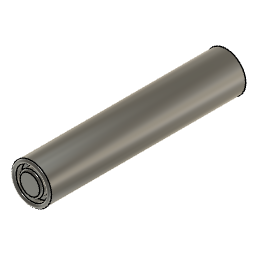
Shaker v1 (Autodesk Fusion 360 archive; units mm, degrees)
design "Shacker Pin Small"
Autodesk Fusion 360 part; units mm, degrees
sketch "Sketch1" plane through (0, 0, 0) normal (0, 1, 0) x (1, 0, 0)
  circle A0 centre (0, 0) radius 5
  dimension "d1" = 10
  constraint coincident A0.centre origin
  measures "d1" diameter of A0
extrude "Extrude1" add sketch "Sketch1" along normal blind 50
sketch "Sketch2" plane through (0, 0, 0) normal (0, -1, 0) x (1, 0, 0)
  circle A0 centre (0, 0) radius 5
  circle A1 centre (0, 0) radius 3
  circle A2 centre (0, 0) radius 4
  dimension "d4" = 6
  dimension "d5" = 8
  constraint coincident A0.centre A1.centre
  constraint concentric A1 A2
  measures "d4" diameter of A1
  measures "d5" diameter of A2
extrude "Extrude2" cut sketch "Sketch2" against normal blind 2 contours A2
fillet "Fillet2" radius 0.5 3 edges at (-2.797, 0, -1.0848) (-3.7293, 0, 1.4465) (-4.6616, 0, 1.8081)

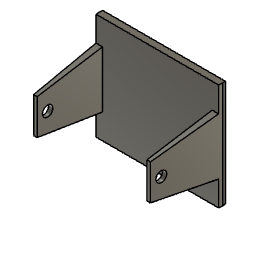
design "Actual Shaker Stand"
Autodesk Fusion 360 part; units mm, degrees
sketch "Sketch1" plane through (0, 0, 0) normal (0, 1, 0) x (1, 0, 0)
  line L0 (0, 0) -> (117.4, 0)
  line L1 (117.4, 0) -> (117.4, -101.6)
  line L2 (117.4, -101.6) -> (0, -101.6)
  line L3 (0, -101.6) -> (0, 0)
  dimension "d1" = 117.4
  dimension "d2" = 101.6
  constraint horizontal L0
  constraint vertical L1
  constraint horizontal L2
  constraint vertical L3
  constraint coincident L0.start L3.end
  measures "d1" distance of L0.start L0.end
  measures "d2" distance of L0.start L2.end
extrude "Extrude1" add sketch "Sketch1" along normal blind 6.35
sketch "Sketch2" plane through (0, 0, 0) normal (0, -1, 0) x (1, 0, 0)
  line L0 (117.4, 101.6) -> (0, 101.6)
  line L1 (0, 101.6) -> (0, 0)
  line L2 (0, 0) -> (117.4, 0)
  line L3 (117.4, 0) -> (117.4, 101.6)
  line L4 (0, 101.6) -> (6.35, 101.6)
  line L5 (0, 0) -> (6.35, 0)
  line L6 (6.35, 101.6) -> (6.35, 0)
  line L7 (0, 0) -> (0, 101.6)
  line L8 (117.4, 0) -> (111.05, 0)
  line L9 (111.05, 0) -> (111.05, 101.6)
  line L10 (117.4, 101.6) -> (117.4, 0)
  dimension "d5" = 6.35
  dimension "d6" = 6.35
  dimension "d7" = 6.35
  constraint coincident L0.end L1.start
  constraint horizontal L4
  constraint coincident L1.end L2.start
  constraint perpendicular L1 L5
  constraint coincident L2.end L3.start
  constraint perpendicular L3 L8
  constraint coincident L0 L9.end
  constraint perpendicular L0 L9
  constraint coincident L0.start L3.end
  measures "d5" distance of L0.end L4.end
  measures "d6" distance of L1.end L5.end
  measures "d7" distance of L2.end L8.end
extrude "Extrude2" add sketch "Sketch2" along normal blind 62.35 contours L0 L2 L3 L8 L9 L10 | L0 L1 L2 L4 L5 L6 L7
sketch "Sketch3" plane through (0, 0, 0) normal (-1, 0, 0) x (0, -1, 0)
  line L0 (62.35, 101.6) -> (-6.35, 101.6)
  line L1 (-6.35, 101.6) -> (-6.35, 0)
  line L2 (-6.35, 0) -> (62.35, 0)
  line L3 (62.35, 0) -> (62.35, 101.6)
  line L4 (-6.35, 101.6) -> (0, 101.6)
  line L5 (0, 0) -> (-6.35, 0)
  line L6 (-6.35, 0) -> (-6.35, 101.6)
  line L7 (62.35, 67.73) -> (62.35, 33.87)
  line L8 (0, 101.6) -> (0, 77.73)
  line L9 (0, 0) -> (0, 23.87)
  line L10 (0, 23.87) -> (62.35, 33.87)
  line L11 (0, 77.73) -> (62.35, 67.73)
  line L12 (0, 77.73) -> (0, 23.87)
  dimension "d10" = 6.35
  dimension "d13" = 23.87
  dimension "d14" = 23.87
  constraint coincident L0.end L1.start
  constraint perpendicular L1 L4
  constraint coincident L5.start L9.start
  constraint coincident L1.end L2.start
  constraint coincident L3 L7.start
  constraint coincident L3 L7.end
  constraint perpendicular L4 L8
  constraint perpendicular L5 L9
  measures "d10" distance of L0.end L4.end
  measures "d13" distance of L4.end L8.end
  measures "d14" distance of L5.start L9.end
extrude "Extrude3" cut sketch "Sketch3" against normal blind 200 contours L0 L3 L8 L11 | L2 L3 L9 L10
sketch "Sketch4" plane through (0, 0, 0) normal (-1, 0, 0) x (0, -1, 0)
  line L0 (62.35, 67.73) -> (0, 77.73)
  line L1 (0, 77.73) -> (0, 101.6)
  line L2 (0, 101.6) -> (-6.35, 101.6)
  line L3 (-6.35, 101.6) -> (-6.35, 0)
  line L4 (-6.35, 0) -> (0, 0)
  line L5 (0, 0) -> (0, 23.87)
  line L6 (0, 23.87) -> (62.35, 33.87)
  line L7 (62.35, 33.87) -> (62.35, 67.73)
  line L8 (62.35, 50.8) -> (52.35, 50.8)
  circle A0 centre (52.35, 50.8) radius 5
  dimension "d17" = 10
  dimension "d18" = 10
  constraint midpoint L7 L8.start
  constraint perpendicular L7 L8
  constraint coincident L8.end A0.centre
  measures "d17" distance of L8.start L8.end
  measures "d18" diameter of A0
extrude "Extrude4" cut sketch "Sketch4" against normal blind 200 contours A0
chamfer "Chamfer1" distance 3 angle 87.4 2 edges at (0, -62.35, 50.8) (117.4, -62.35, 50.8) measured on face at (2.1167, -62.35, 56.4433) measured on face at (113.1667, -62.35, 45.1567)
